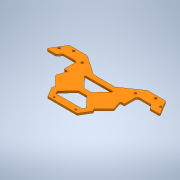
# Autodesk Inventor part: RCT-H001_Al_side_plate
Saved by Autodesk Inventor 2020 (Build 240168000, 168)
## iProperties
Created: 2019-09-17
Part Number: RCT-H001_Al_side_plate
Material: Generic
Document SubType Name: Modeling
Designer: maste
Density: 1 g/cm^3
Appearance: Orange
Author: maste
Autodesk Inventor part; units mm, degrees
ref_plane "YZ Plane" through (0, 0, 0) normal (1, 0, 0) x (0, 1, 0)
ref_plane "XZ Plane" through (0, 0, 0) normal (0, 1, 0) x (-1, 0, 0)
ref_plane "XY Plane" through (0, 0, 0) normal (0, 0, 1) x (1, 0, 0)
sketch "Sketch1" plane through (0, 0, 0) normal (0, 0, 1) x (1, 0, 0)
  line L0 (0, 76.5) -> (84, 76.5) construction
  line L1 (84, 76.5) -> (84, 0) construction
  line L2 (84, 0) -> (0, 0) construction
  line L3 (0, 0) -> (0, 76.5) construction
  line L4 (-37, 76.5) -> (0, 76.5) construction
  line L5 (0, 76.5) -> (0, 62) construction
  line L6 (0, 62) -> (-37, 62) construction
  line L7 (-37, 62) -> (-37, 76.5) construction
  line L8 (84, 76.5) -> (121, 76.5) construction
  line L9 (121, 76.5) -> (121, 62) construction
  line L10 (121, 62) -> (84, 62) construction
  line L11 (84, 62) -> (84, 76.5) construction
  line L12 (27, 58) -> (57, 58)
  line L13 (27, 58) -> (0.7665, 75.9748)
  line L14 (57, 58) -> (83.2335, 75.9748)
  line L15 (13.25, 14) -> (70.75, 14) construction
  line L16 (0, 76.5) -> (-25, 76.5) construction
  line L17 (-37, 76.5) -> (-37, 56.5) construction
  line L18 (-36.0913, 58.0145) -> (-25.5826, 75.529)
  line L19 (-35.2338, 56.5) -> (-23.9739, 56.5)
  line L20 (0, 62) -> (-19, 62) construction
  line L21 (-19.6002, 61.2665) -> (-23.1999, 56.8668)
  line L22 (0, 44) -> (84, 44) construction
  line L23 (1, 44) -> (4.371, 44)
  line L24 (83, 44) -> (79.629, 44)
  line L25 (1.5, 31) -> (82.5, 31) construction
  line L26 (5.3215, 42.6893) -> (1.6893, 31.579)
  line L27 (78.6785, 42.6893) -> (82.3107, 31.579)
  line L28 (15.3, 17) -> (68.7, 17) construction
  line L29 (82.0724, 30.5662) -> (69.278, 17.5864)
  line L30 (1.9276, 30.5662) -> (14.722, 17.5864)
  line L31 (69.1645, 16.3202) -> (70.3916, 14.5245)
  line L32 (14.8355, 16.3202) -> (13.6084, 14.5245)
  line L33 (21.5, 0) -> (62.5, 0) construction
  line L34 (21.2099, 0.4923) -> (13.5725, 13.4527)
  line L35 (62.7901, 0.4923) -> (70.4275, 13.4527)
  line L36 (84, 76.5) -> (109, 76.5) construction
  line L37 (121, 76.5) -> (121, 56.5) construction
  line L38 (120.0913, 58.0145) -> (109.5826, 75.529)
  line L39 (119.2338, 56.5) -> (107.9739, 56.5)
  line L40 (84, 62) -> (103, 62) construction
  line L41 (103.6002, 61.2665) -> (107.1999, 56.8668)
  line L42 (-23.8676, 76.5) -> (-0.9292, 76.5)
  line L43 (84.9292, 76.5) -> (107.8676, 76.5)
  line L44 (-18.0522, 62) -> (-2, 62)
  line L45 (102.0522, 62) -> (86, 62)
  line L46 (0, 60) -> (0, 45)
  line L47 (84, 60) -> (84, 45)
  line L48 (22.0714, 0) -> (61.9286, 0)
  line L49 (23.861, 51) -> (60.139, 51)
  line L50 (37.4235, 35) -> (46.5765, 35)
  line L51 (47.2947, 35.3042) -> (60.8572, 49.3042)
  line L52 (36.7053, 35.3042) -> (23.1428, 49.3042)
  line L53 (36.4346, 28) -> (47.5654, 28)
  line L54 (22, 13) -> (62, 13) construction
  line L55 (24.193, 9) -> (59.807, 9)
  line L56 (60.7433, 9.6489) -> (61.7824, 12.4197)
  line L57 (61.5771, 13.4531) -> (48.2965, 27.6823)
  line L58 (35.7035, 27.6823) -> (22.4229, 13.4531)
  line L59 (22.2176, 12.4197) -> (23.2567, 9.6489)
  line L60 (-28.5, 66) -> (112.5, 66) construction
  line L61 (-15, 72.5) -> (99, 72.5) construction
  line L62 (27, 3.5) -> (57, 3.5) construction
  arc A0 (0.7665, 75.9748) -> (-0.9292, 76.5) centre (-0.9292, 73.5) ccw
  arc A1 (84.9292, 76.5) -> (83.2335, 75.9748) centre (84.9292, 73.5) ccw
  arc A2 (-23.8676, 76.5) -> (-25.5826, 75.529) centre (-23.8676, 74.5) ccw
  arc A3 (109.5826, 75.529) -> (107.8676, 76.5) centre (107.8676, 74.5) ccw
  arc A4 (119.2338, 56.5) -> (120.0913, 58.0145) centre (119.2338, 57.5) ccw
  arc A5 (-36.0913, 58.0145) -> (-35.2338, 56.5) centre (-35.2338, 57.5) ccw
  arc A6 (-23.9739, 56.5) -> (-23.1999, 56.8668) centre (-23.9739, 57.5) ccw
  arc A7 (107.1999, 56.8668) -> (107.9739, 56.5) centre (107.9739, 57.5) ccw
  arc A8 (103.6002, 61.2665) -> (102.0522, 62) centre (102.0522, 60) ccw
  arc A9 (-18.0522, 62) -> (-19.6002, 61.2665) centre (-18.0522, 60) ccw
  line L63 (-2, 62) -> (0, 60)
  line L64 (84, 60) -> (86, 62)
  arc A10 (0, 45) -> (1, 44) centre (1, 45) ccw
  arc A11 (83, 44) -> (84, 45) centre (83, 45) ccw
  arc A12 (79.629, 44) -> (78.6785, 42.6893) centre (79.629, 43) ccw
  arc A13 (5.3215, 42.6893) -> (4.371, 44) centre (4.371, 43) ccw
  arc A14 (1.6893, 31.579) -> (1.9276, 30.5662) centre (2.6398, 31.2682) ccw
  arc A15 (82.0724, 30.5662) -> (82.3107, 31.579) centre (81.3602, 31.2682) ccw
  arc A16 (69.278, 17.5864) -> (69.1645, 16.3202) centre (69.9902, 16.8844) ccw
  arc A17 (70.4275, 13.4527) -> (70.3916, 14.5245) centre (69.5659, 13.9603) ccw
  arc A18 (61.9286, 0) -> (62.7901, 0.4923) centre (61.9286, 1) ccw
  arc A19 (21.2099, 0.4923) -> (22.0714, 0) centre (22.0714, 1) ccw
  arc A20 (13.6084, 14.5245) -> (13.5725, 13.4527) centre (14.4341, 13.9603) ccw
  arc A21 (14.8355, 16.3202) -> (14.722, 17.5864) centre (14.0098, 16.8844) ccw
  arc A22 (23.2567, 9.6489) -> (24.193, 9) centre (24.193, 10) ccw
  arc A23 (22.4229, 13.4531) -> (22.2176, 12.4197) centre (23.154, 12.7708) ccw
  arc A24 (36.4346, 28) -> (35.7035, 27.6823) centre (36.4346, 27) ccw
  arc A25 (48.2965, 27.6823) -> (47.5654, 28) centre (47.5654, 27) ccw
  arc A26 (61.7824, 12.4197) -> (61.5771, 13.4531) centre (60.846, 12.7708) ccw
  arc A27 (59.807, 9) -> (60.7433, 9.6489) centre (59.807, 10) ccw
  arc A28 (23.861, 51) -> (23.1428, 49.3042) centre (23.861, 50) ccw
  arc A29 (60.8572, 49.3042) -> (60.139, 51) centre (60.139, 50) ccw
  arc A30 (46.5765, 35) -> (47.2947, 35.3042) centre (46.5765, 36) ccw
  arc A31 (36.7053, 35.3042) -> (37.4235, 35) centre (37.4235, 36) ccw
  circle A32 centre (-15, 72.5) radius 1.5
  circle A33 centre (-28.5, 66) radius 1.5
  circle A34 centre (112.5, 66) radius 1.5
  circle A35 centre (99, 72.5) radius 1.5
  circle A36 centre (57, 3.5) radius 1.25
  circle A37 centre (27, 3.5) radius 1.25
  line L65 (5, 64.5) -> (79, 64.5) construction
  circle A38 centre (5, 64.5) radius 1.5
  circle A39 centre (79, 64.5) radius 1.5
  point P0 (-23.5, 56.5)
  point P1 (5.75, 44)
  point P2 (78.25, 44)
  point P3 (107.5, 56.5)
  point P4 (21.5, 51)
  point P5 (62.5, 51)
  point P6 (37, 35)
  point P7 (47, 35)
  point P8 (36, 28)
  point P9 (48, 28)
  point P10 (23.5, 9)
  point P11 (60.5, 9)
  dimension "d0" = 84
  dimension "d1" = 76.5
  dimension "d2" = 37
  dimension "d3" = 14.5
  dimension "d4" = 14.5
  dimension "d5" = 37
  dimension "d7" = 30
  dimension "d8" = 27
  dimension "d9" = 58
  dimension "d10" = 57.5
  dimension "d11" = 13.25
  dimension "d12" = 14
  dimension "d13" = 25
  dimension "d14" = 20
  dimension "d15" = 13.5
  dimension "d16" = 19
  dimension "d17" = 18
  dimension "d18" = 5.75
  dimension "d19" = 5.75
  dimension "d20" = 81
  dimension "d21" = 13
  dimension "d22" = 1.5
  dimension "d23" = 53.4
  dimension "d24" = 14
  dimension "d25" = 15.3
  dimension "d26" = 41
  dimension "d27" = 21.5
  dimension "d28" = 25
  dimension "d29" = 20
  dimension "d30" = 13.5
  dimension "d31" = 19
  dimension "d32" = 41
  dimension "d33" = 21.5
  dimension "d34" = 7
  dimension "d35" = 10
  dimension "d36" = 23
  dimension "d37" = 37
  dimension "d38" = 12
  dimension "d39" = 28
  dimension "d40" = 36
  dimension "d41" = 40
  dimension "d42" = 13
  dimension "d43" = 22
  dimension "d44" = 37
  dimension "d45" = 9
  dimension "d46" = 23.5
  dimension "d47" = 141
  dimension "d48" = 10.5
  dimension "d49" = 8.5
  dimension "d50" = 114
  dimension "d51" = 4
  dimension "d52" = 22
  dimension "d53" = 30
  dimension "d54" = 3.5
  dimension "d55" = 27
  dimension "d56" = 3
  dimension "d57" = 3
  dimension "d58" = 2
  dimension "d59" = 2
  dimension "d60" = 1
  dimension "d61" = 1
  dimension "d62" = 1
  dimension "d63" = 1
  dimension "d64" = 2
  constraints: 132 end point, 78 point on line, 64 point on circle, 64 tangent, 40 centre point, 19 horizontal, 17 equal radius, 15 coincident, 6 parallel, 5 collinear, 4 perpendicular, 3 vertical
  measures "d0" distance of L0.start L0.end
  measures "d1" distance of L2.end L0.start
  measures "d2" distance of L0.start L4.start
  measures "d3" distance of L6.end L4.start
  measures "d4" distance of L0.end L10.end
  measures "d5" distance of L0.end L8.end
  measures "d7" distance of L12.start L12.end
  measures "d8" distance from line of L3 L12.start
  measures "d9" distance between parallel lines of L2 L12
  measures "d10" distance of L15.start L15.end
  measures "d11" distance from line of L3 L15.start
  measures "d12" distance between parallel lines of L2 L15
  measures "d13" distance of L0.start L16.end
  measures "d14" distance of L4.start L17.end
  measures "d15" distance of L17.end point (-23.5, 56.5)
  measures "d16" distance of L5.end L20.end
  measures "d17" distance between parallel lines of L10 L22
  measures "d18" distance of L22.start point (5.75, 44)
  measures "d19" distance of L22.end point (78.25, 44)
  measures "d20" distance of L25.start L25.end
  measures "d21" distance between parallel lines of L22 L25
  measures "d22" distance from line of L3 L25.start
  measures "d23" distance of L28.start L28.end
  measures "d24" distance between parallel lines of L25 L28
  measures "d25" distance from line of L3 L28.start
  measures "d26" distance of L33.start L33.end
  measures "d27" distance from line of L3 L33.start
  measures "d28" distance of L0.end L36.end
  measures "d29" distance of L8.end L37.end
  measures "d30" distance of L37.end point (107.5, 56.5)
  measures "d31" distance of L10.end L40.end
  measures "d32" distance of point (21.5, 51) point (62.5, 51)
  measures "d33" distance from line of L46 point (21.5, 51)
  measures "d34" distance between parallel lines of L49 L12
  measures "d35" distance of point (37, 35) point (47, 35)
  measures "d36" distance between parallel lines of L12 L50
  measures "d37" distance from line of L3 point (37, 35)
  measures "d38" distance of point (36, 28) point (48, 28)
  measures "d39" distance between parallel lines of L33 L53
  measures "d40" distance from line of L3 point (36, 28)
  measures "d41" distance of L54.start L54.end
  measures "d42" distance between parallel lines of L2 L54
  measures "d43" distance from line of L3 L54.start
  measures "d44" distance of point (23.5, 9) point (60.5, 9)
  measures "d45" distance between parallel lines of L2 L55
  measures "d46" distance from line of L3 point (23.5, 9)
  measures "d47" distance of L60.start L60.end
  measures "d48" distance between parallel lines of L60 L0
  measures "d49" horizontal distance of L17.end L60.start
  measures "d50" distance of L61.start L61.end
  measures "d51" distance between parallel lines of L16 L61
  measures "d52" horizontal distance of L17.end L61.start
  measures "d53" distance of L62.start L62.end
  measures "d54" distance between parallel lines of L2 L62
  measures "d55" distance from line of L3 L62.start
  measures "d56" radius of A0
  measures "d57" radius of A1
  measures "d58" radius of A2
  measures "d59" radius of A3
  measures "d60" radius of A4
  measures "d61" radius of A5
  measures "d62" radius of A6
  measures "d63" radius of A7
  measures "d64" radius of A8
extrude "Extrusion3" add sketch "Sketch1" along normal blind 2.5
body "Solid3"
